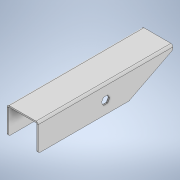
# Autodesk Inventor part: pedalDer
Saved by Autodesk Inventor 2021.2 (Build 252289000, 289)
## iProperties
Created: 2026-06-16
Part Number: pedalDer
Material: Generic
Document SubType Name: Sheet Metal
Designer: nelso
Density: 1 g/cm^3
Sheet Metal Rule: Default_mm
Appearance: Default
Author: nelso
Autodesk Inventor part; units mm, degrees
ref_plane "YZ Plane" through (0, 0, 0) normal (1, 0, 0) x (0, 1, 0)
ref_plane "XZ Plane" through (0, 0, 0) normal (0, 1, 0) x (-1, 0, 0)
ref_plane "XY Plane" through (0, 0, 0) normal (0, 0, 1) x (1, 0, 0)
sketch "Sketch1" plane through (0, 0, 0) normal (0, 1, 0) x (-1, 0, 0)
  line L0 (-30, -150) -> (30, -150)
  line L1 (30, -150) -> (30, 150)
  line L2 (30, 150) -> (-30, 150)
  line L3 (-30, 150) -> (-30, -150)
  line L4 (-30, -150) -> (30, 150) construction
  line L5 (30, -150) -> (-30, 150) construction
  line L6 (30, 0) -> (30, 40)
  line L7 (30, 0) -> (30, -25)
  line L8 (-30, -150) -> (0, -150)
  line L9 (-30, -150) -> (30, -150)
  line L10 (30, -25) -> (30, -150)
  line L11 (30, 40) -> (40, 150)
  point P0 (0, 0)
  dimension "d0" = 60
  dimension "d1" = 300
  dimension "d2" = 40
  dimension "d3" = 25
  dimension "d5" = 60
  dimension "d6" = 70
  measures "d0" distance of L2.end L1.end
  measures "d1" distance of L1.end L0.end
  measures "d2" distance of L6.start L6.end
  measures "d3" distance of L6.start L7.end
  measures "d5" distance of L9.end L0.start
  measures "d6" distance of L11.end L2.end
extrude "Plate1" add sketch "Sketch1" along normal blind 3.1
sketch "Sketch2" plane through (31.516, -1.516, 150) normal (1, 0, 0) x (0, 1, 0)
  line L0 (0, -300) -> (0, 0)
  line L1 (0, 0) -> (-55.384, 0)
  line L2 (-55.384, 0) -> (-55.384, -300)
  line L3 (-55.384, -300) -> (0, -300)
  constraints: 6 end point, 1 horizontal, 1 perpendicular, 1 vertical
edge flange "Flange1" height 60 angle 90 thickness 3.1 bend radius 1.516 thickness toward (1, 0, 0) relief straight relief width 3.1 relief depth 1.55 corner gap 1.516 corner form 0 edges at (30, 0, 0) (-30, 0, 95) (-30, 0, 20) (-30, 0, -12.5) (-30, 0, -87.5) wall of the first edge with corners at (31.516, -1.516, -150) (31.516, -1.516, 150) (31.516, -56.9, 150) (31.516, -56.9, -150)
bend "Bend1"
corner "Corner1"
sketch "Sketch5" plane through (34.616, -56.9, 150) normal (1, 0, 0) x (0, 0, -1)
  line L0 (140.7624, 27.692) -> (145.3812, 35.692)
  line L1 (145.3812, 35.692) -> (154.6188, 35.692)
  line L2 (154.6188, 35.692) -> (159.2376, 27.692)
  line L3 (159.2376, 27.692) -> (154.6188, 19.692)
  line L4 (154.6188, 19.692) -> (145.3812, 19.692)
  line L5 (145.3812, 19.692) -> (140.7624, 27.692)
  line L6 (0, 60) -> (300, 60) projected
  line L7 (0, 60) -> (0, 50)
  line L8 (0, 0) -> (0, 55.384) projected
  line L9 (0, 50) -> (97.9796, 0)
  line L10 (300, 0) -> (0, 0) projected
  line L11 (150, 0) -> (202.2, 0)
  line L12 (202.2, 0) -> (300, 50)
  line L13 (300, 0) -> (300, 55.384) projected
  point P0 (150, 56.9)
  point P1 (150, 27.692)
  dimension "d35" = 16
  dimension "d38" = 10
  dimension "d39" = 110
  dimension "d40" = 52.2
  constraints: 20 end point, 4 point on line, 1 midpoint, 13 other
  measures "d35" distance between parallel lines of L4 L1
  measures "d38" distance of L6.start L7.end
  measures "d39" distance of L7.end L9.end
  measures "d40" distance of L11.start L11.end
extrude "Cut3" cut sketch "Sketch5" against normal through all contours L0 L1 L2 L3 L4 L5 | L8 L9 L10
mirror "Mirror2" about plane through (0, 0, 0) normal (0, 0, 1) remove original yes
fillet "Corner Round2" radius 4 6 edges at (-33.066, -6.9, -150) (-33.066, -56.9, -52.0204) (33.066, -6.9, -150) (33.066, -56.9, -52.0204) (33.066, -56.9, 150) (-33.066, -56.9, 150)
equation "\"d36\" = Thickness"
equation "\"d7\" = Thickness"
equation "\"d8\" = BendReliefWidth"
equation "\"d9\" = BendReliefDepth"
equation "\"d10\" = MinimumRemnant"
equation "\"d11\" = TransitionRadius"
equation "\"d14\" = BendRadius"
equation "\"d15\" = CornerReliefSize"
equation "\"d16\" = GapSize"
equation "\"d17\" = JacobiRadiusSize"
equation "\"BendReliefWidth\" = Thickness"
equation "\"BendReliefDepth\" = 0.5 * Thickness"
equation "\"CornerReliefSize\" = 4 * Thickness"
equation "\"MinimumRemnant\" = 2 * Thickness"
equation "\"TransitionRadius\" = BendRadius"
equation "\"JacobiRadiusSize\" = BendRadius"
equation "\"GapSize\" = Thickness"
equation "\"Thickness\" = 3.1"
equation "\"BendRadius\" = 1.516"
body "Solid1"
